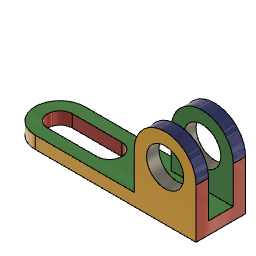
Exercise 5 IRFAN NAUFAL Calameo v2 (Autodesk Fusion 360 design; units mm, degrees)
Autodesk Fusion 360 part; units mm, degrees
sketch "Sketch1" plane through (0, 0, 0) normal (0, 0, 1) x (1, 0, 0)
  line L0 (0, 0) -> (40, 0)
  line L1 (40, 40) -> (0, 40)
  line L2 (40, 40) -> (105, 40)
  line L3 (105, 0) -> (40, 0)
  line L4 (105, 40) -> (130, 40)
  line L5 (130, 40) -> (130, 0)
  line L6 (130, 0) -> (105, 0)
  line L7 (0, 30) -> (40, 30)
  line L8 (0, 10) -> (40, 10)
  arc A0 (40, 10) -> (40, 30) centre (40, 20) ccw
  arc A1 (0, 30) -> (0, 10) centre (0, 20) ccw
  arc A2 (0, 40) -> (0, 0) centre (0, 20) ccw
  line L9 (130, 40) -> (80, 40)
  line L10 (80, 40) -> (80, 30)
  line L11 (80, 30) -> (130, 30)
  line L12 (130, 30) -> (130, 40)
  line L13 (130, 0) -> (80, 0)
  line L14 (80, 0) -> (80, 10)
  line L15 (80, 10) -> (130, 10)
  line L16 (130, 10) -> (130, 0)
  dimension "d1" = 40
  dimension "d2" = 40
  dimension "d3" = 65
  dimension "d4" = 40
  dimension "d5" = 25
  dimension "d6" = 40
  dimension "d8" = 20
  dimension "d9" = 40
  dimension "d10" = 20
  dimension "d11" = 50
  dimension "d12" = 10
  dimension "d13" = 50
  dimension "d14" = 10
  constraint horizontal L0
  constraint horizontal L1
  constraint coincident L0.start A2.end
  constraint horizontal L2
  constraint horizontal L3
  constraint horizontal L4
  constraint vertical L5
  constraint horizontal L6
  constraint concentric A1 A2
  constraint horizontal L9
  constraint vertical L10
  constraint horizontal L11
  constraint vertical L12
  constraint horizontal L13
  constraint vertical L14
  constraint horizontal L15
  constraint vertical L16
  measures "d1" distance of L0.start L0.end
  measures "d2" distance of L0.start L1.end
  measures "d3" distance of L1.start L2.end
  measures "d4" distance of L1.start L0.end
  measures "d5" distance of L2.end L4.end
  measures "d6" distance of L2.end L3.start
  measures "d8" diameter of A1
  measures "d9" diameter of A2
  measures "d10" diameter of A0
  measures "d11" distance of L4.end L9.end
  measures "d12" distance of L4.end L11.end
  measures "d13" distance of L5.end L13.end
  measures "d14" distance of L5.end L15.end
extrude "Extrude1" add sketch "Sketch1" along normal blind 10 contours L0 L1 L2 L3 L5 A2 L10 L11 L14 L15
extrude "Extrude2" add sketch "Sketch1" along normal blind 65 contours L3 L5 L6 L13 L14 L15 L16 | L2 L4 L5 L9 L10 L11 L12
sketch "Sketch2" plane through (0, 0, 0) normal (0, -1, 0) x (1, 0, 0)
  line L0 (0, 0) -> (130, 0)
  line L1 (130, 0) -> (130, 65)
  line L2 (80, 65) -> (80, 10)
  line L3 (80, 10) -> (0, 10)
  line L4 (0, 10) -> (0, 0)
  line L5 (130, 0) -> (130, 40)
  line L6 (130, 40) -> (80, 40)
  circle A0 centre (105, 40) radius 15
  circle A1 centre (105, 40) radius 25
  dimension "d19" = 40
  dimension "d20" = 30
  constraint coincident L0.end L1.start
  constraint coincident L1 L5.end
  constraint coincident L2 L6.end
  constraint perpendicular L2 L6
  constraint midpoint L6 A0.centre
  constraint concentric A0 A1
  measures "d19" distance of L0.end L5.end
  measures "d20" diameter of A0
extrude "Extrude3" cut sketch "Sketch2" against normal blind 55 contours L6 A0 | L6 A0
extrude "Extrude4" add sketch "Sketch2" along normal blind 9 contours L6 A0 A1 picked at (95.2888, 59.3043)
extrude "Extrude5" cut 2 faces at (125.0884, 0, 60.0884) (84.9116, 0, 60.0884) along direction (0, 1, 0) blind 57
extrude "Extrude6" cut 1 faces at (95.2888, -9, 59.3043) along direction (0, 1, 0) blind 9
